Autodesk Fusion 360 part; units mm, degrees
note: some values were not read from the file. Chosen so that the rebuilt part matches the saved one: a direction; which face or edge a step refers to; that a step has no effect; which pieces of a blend or face edit are solid. Set by a fixed rule: which sketch regions a step uses.
(part 2 of 2)
sketch "Esquisse54" plane through (0, 0, 0) normal (0, 0, 1) x (1, 0, 0)
  line L0 (-107.000002, 15) -> (-127.000002, 15)
  line L1 (-129.000002, 17) -> (-129.000002, 37)
  line L2 (-127.000002, 39) -> (-107.000002, 39)
  line L3 (-105.000002, 37) -> (-105.000002, 17)
  arc A0 (-107.000002, 15) -> (-105.000002, 17) centre (-107.000002, 17) ccw
  arc A1 (-129.000002, 17) -> (-127.000002, 15) centre (-127.000002, 17) ccw
  arc A2 (-127.000002, 39) -> (-129.000002, 37) centre (-127.000002, 37) ccw
  arc A3 (-105.000002, 37) -> (-107.000002, 39) centre (-107.000002, 37) ccw
  point P0 (-105.000002, 15)
  point P1 (-129.000002, 15)
  point P2 (-105.000002, 39)
  dimension "d387" = 24
  dimension "d388" = 24
  dimension "d389" = 2
  constraint horizontal L0
  constraint vertical L1
  constraint horizontal L2
  constraint vertical L3
  constraint tangent L0 A0
  constraint tangent L3 A0
  constraint tangent L0 A1
  constraint tangent L1 A1
  constraint equal A0 A1
  constraint tangent L1 A2
  constraint tangent L2 A2
  constraint equal A0 A2
  constraint tangent L2 A3
  constraint tangent L3 A3
  constraint equal A0 A3
  measures "d389" radius of A0
extrude "Extrusion54" add sketch "Esquisse54" along normal blind 2.5 separate body makes body 8
sketch "Esquisse55" plane through (0, 0, 2.5) normal (0, 0, 1) x (-1, 0, 0)
  arc A0 (107.000002, -15) -> (105.000002, -17) centre (107.000002, -17) ccw
  line L0 (105.000002, -17) -> (105.000002, -37)
  arc A1 (105.000002, -37) -> (107.000002, -39) centre (107.000002, -37) ccw
  line L1 (107.000002, -39) -> (127.000002, -39)
  arc A2 (127.000002, -39) -> (129.000002, -37) centre (127.000002, -37) ccw
  line L2 (129.000002, -37) -> (129.000002, -17)
  arc A3 (129.000002, -17) -> (127.000002, -15) centre (127.000002, -17) ccw
  line L3 (127.000002, -15) -> (107.000002, -15)
  line L4 (117.000002, -39) -> (117.000002, -15)
  line L5 (117.000002, -39) -> (117.000002, -33)
  line L6 (117.000002, -39) -> (117.000002, -33)
  line L7 (117.000002, -33) -> (114.000002, -33)
  line L8 (114.000002, -33) -> (120.000002, -33)
  line L9 (120.000002, -33) -> (120.000002, -42)
  line L10 (120.000002, -42) -> (114.000002, -42)
  line L11 (114.000002, -42) -> (114.000002, -33)
  line L12 (117.000002, -15) -> (117.000002, -21)
  line L13 (117.000002, -21) -> (114.000002, -21)
  line L14 (114.000002, -21) -> (120.000002, -21)
  line L15 (120.000002, -21) -> (120.000002, -11)
  line L16 (120.000002, -11) -> (114.000002, -11)
  line L17 (114.000002, -11) -> (114.000002, -21)
  dimension "d392" = 3
  dimension "d393" = 6
  dimension "d394" = 9
  dimension "d395" = 6
  dimension "d396" = 3
  constraint perpendicular L1 L6
  constraint perpendicular L5 L7
  constraint horizontal L8
  constraint vertical L9
  constraint horizontal L10
  constraint vertical L11
  constraint perpendicular L3 L12
  constraint perpendicular L4 L13
  constraint horizontal L14
  constraint vertical L15
  constraint horizontal L16
  constraint vertical L17
extrude "Extrusion55" add sketch "Esquisse55" along normal blind 2 contours L3 L15 L16 L17 | L3 L4 L12 L13 L14 L17 | L3 L4 L12 L14 L15 | L1 L4 L5 L6 L7 L8 L11 | L1 L9 L10 L11 | L1 L4 L5 L6 L8 L9 picked at (117.000002, -12.333334) picked at (116.000002, -17) picked at (118.000002, -19) picked at (115.000002, -37) picked at (117.000002, -41) picked at (118.000002, -35) bodies 8
fillet "Congé24" radius 5.5 6 edges at (-117.000002, 33, 2.5) (-120.000002, 36, 2.5) (-120.000002, 18, 2.5) (-114.000002, 36, 2.5) (-114.000002, 18, 2.5) (-117.000002, 21, 2.5) on bodies 8
fillet "Congé25" radius 1 4 edges at (-114.000002, 42, 3.5) (-120.000002, 42, 3.5) (-120.000002, 11, 3.5) (-114.000002, 11, 3.5) on bodies 8
sketch "Esquisse56" plane through (0, 0, 4.986655) normal (0, 0, -1) x (1, 0, 0)
  circle A0 centre (15.050001, -71.849998) radius 1.775
  line L0 (4.05, -76.15) -> (4.05, -2.05)
  line L1 (4.05, -2.05) -> (45.95, -2.05)
  line L2 (45.95, -2.05) -> (45.95, -76.15)
  line L3 (45.95, -76.15) -> (39.45, -76.15)
  arc A1 (37.95, -74.65) -> (39.45, -76.15) centre (39.45, -74.65) ccw
  line L4 (37.95, -74.65) -> (37.95, -69.05)
  arc A2 (39.45, -67.55) -> (37.95, -69.05) centre (39.45, -69.05) ccw
  line L5 (39.45, -67.55) -> (45.05, -67.55)
  line L6 (45.05, -67.55) -> (45.05, -10.05)
  line L7 (45.05, -10.05) -> (39.45, -10.05)
  arc A3 (37.95, -8.55) -> (39.45, -10.05) centre (39.45, -8.55) ccw
  line L8 (37.95, -8.55) -> (37.95, -2.950001)
  line L9 (37.95, -2.950001) -> (12.05, -2.950001)
  line L10 (12.05, -2.950001) -> (12.05, -8.55)
  arc A4 (10.55, -10.05) -> (12.05, -8.55) centre (10.55, -8.55) ccw
  line L11 (10.55, -10.05) -> (4.95, -10.05)
  line L12 (4.95, -10.05) -> (4.95, -67.55)
  line L13 (4.95, -67.55) -> (10.55, -67.55)
  arc A5 (12.05, -69.05) -> (10.55, -67.55) centre (10.55, -69.05) ccw
  line L14 (12.05, -69.05) -> (12.05, -74.65)
  arc A6 (10.55, -76.15) -> (12.05, -74.65) centre (10.55, -74.65) ccw
  line L15 (10.55, -76.15) -> (4.05, -76.15)
  arc A7 (5.5, 0) -> (2, -3.5) centre (5.5, -3.5) ccw
  line L16 (2, -3.5) -> (2, -77.731732)
  arc A8 (2, -77.731732) -> (5.5, -81.231732) centre (5.5, -77.731732) ccw
  line L17 (5.5, -81.231732) -> (44.5, -81.231732)
  arc A9 (44.5, -81.231732) -> (48, -77.731732) centre (44.5, -77.731732) ccw
  line L18 (48, -77.731732) -> (48, -3.5)
  arc A10 (48, -3.5) -> (44.5, 0) centre (44.5, -3.5) ccw
  line L19 (44.5, 0) -> (5.5, 0)
  circle A11 centre (34.449701, -71.85) radius 1.25
  dimension "d403" = 2.5
  measures "d403" diameter of A11
extrude "Extrusion56" cut sketch "Esquisse56" against normal blind 3 contours A11 picked at (34.105435, -72.208919) bodies 5
sketch "Esquisse57" plane through (-65, 0, 0) normal (-1, 0, 0) x (0, -1, 0)
  line L0 (-72.369938, 16.885532) -> (-77.56955, 0)
  line L1 (-77.56955, 0) -> (-3.5, 0)
  line L2 (-3.5, 0) -> (-3.5, 12.67458)
  arc A0 (-3.5, 12.67458) -> (-4.57746, 17.53469) centre (-15, 12.67458) ccw
  line L3 (-4.57746, 17.53469) -> (-10.929276, 31.156202)
  arc A1 (-10.929276, 31.156202) -> (-13.220087, 34.42782) centre (-21.351815, 26.296092) ccw
  line L4 (-13.220087, 34.42782) -> (-17.197997, 38.405729)
  arc A2 (-17.197997, 38.405729) -> (-23.332771, 41.59929) centre (-25.329725, 30.274001) ccw
  line L5 (-23.332771, 41.59929) -> (-27.862877, 42.39807)
  arc A3 (-27.862877, 42.39807) -> (-33.577928, 40.866727) centre (-29.078415, 35.504416) ccw
  line L6 (-33.577928, 40.866727) -> (-58.168726, 20.232597)
  line L7 (-58.168726, 20.232597) -> (-70.308204, 18.628242)
  arc A4 (-70.308204, 18.628242) -> (-72.369938, 16.885532) centre (-69.980652, 16.149793) ccw
  circle A5 centre (-60.783686, 14.226399) radius 3
  dimension "d406" = 6
  measures "d406" diameter of A5
extrude "Extrusion57" cut sketch "Esquisse57" against normal blind 7 contours A5 picked at (-61.223757, 16.154477) bodies 1
equation "d305 = Diametre_canne"
equation "Diametre_canne = 13.30 mm"
named bodies: "Body1", "Body2"
